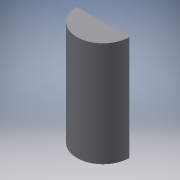
# Autodesk Inventor part: Part44
Saved by Autodesk Inventor 2016 (Build 200138000, 138)
## iProperties
Created: 2016-01-27
Part Number: Part44
Material: Generic
Document SubType Name: Modeling
Designer: seve
Density: 1 g/cm^3
Appearance: Default
Author: seve
Autodesk Inventor part; units mm, degrees
ref_plane "YZ Plane" through (0, 0, 0) normal (1, 0, 0) x (0, 1, 0)
ref_plane "XZ Plane" through (0, 0, 0) normal (0, 1, 0) x (-1, 0, 0)
ref_plane "XY Plane" through (0, 0, 0) normal (0, 0, 1) x (1, 0, 0)
sketch "Sketch1" plane through (0, 0, 0) normal (0, 1, 0) x (-1, 0, 0)
  arc A0 (3.175, 0) -> (-3.175, 0) centre (0, 0) ccw
  line L0 (-3.175, -4.7625) -> (-3.175, 0) projected
  line L1 (3.175, -4.7625) -> (3.175, 0) projected
  line L2 (-3.175, 0) -> (3.175, 0)
  constraints: 2 end point, 2 point on circle, 1 centre point, 1 coincident, 1 perpendicular, 1 tangent
extrude "Extrusion1" add sketch "Sketch1" along normal mid plane 12.7
body "Solid1"
